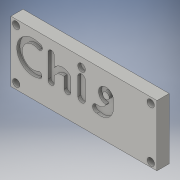
# Autodesk Inventor part: NewName
Saved by Autodesk Inventor 2016 (Build 200138000, 138)
## iProperties
Created: 2016-09-23
Part Number: NewName
Material: Generic
Document SubType Name: Modeling
Designer: Shaan Sharma
Density: 1 g/cm^3
Appearance: Default
Author: Shaan Sharma
Autodesk Inventor part; units mm, degrees
ref_plane "YZ Plane" through (0, 0, 0) normal (1, 0, 0) x (0, 1, 0)
ref_plane "XZ Plane" through (0, 0, 0) normal (0, 1, 0) x (-1, 0, 0)
ref_plane "XY Plane" through (0, 0, 0) normal (0, 0, 1) x (1, 0, 0)
sketch "Sketch1" plane through (0, 0, 0) normal (0, 0, 1) x (1, 0, 0)
  line L0 (-174.625, 111.125) -> (130.175, 111.125)
  line L1 (130.175, 111.125) -> (130.175, -15.875)
  line L2 (130.175, -15.875) -> (-174.625, -15.875)
  line L3 (-174.625, -15.875) -> (-174.625, 111.125)
  point P0 (0, 0)
  dimension "d0" = 127
  dimension "d1" = 304.8
  constraints: 8 end point, 2 parallel, 1 horizontal, 1 perpendicular
  measures "d0" distance of L2.end L0.start
  measures "d1" distance of L1.end L2.end
extrude "Extrusion1" add sketch "Sketch1" along normal blind 25.4
sketch "Sketch2" plane through (0, 0, 25.4) normal (0, 0, 1) x (1, 0, 0)
  arc A0 (-115.8875, 79.375) -> (-115.8875, 41.275) centre (-128.1906, 60.325) ccw
  arc A1 (-115.8875, 92.075) -> (-115.8875, 28.575) centre (-128.1906, 60.325) ccw
  arc A2 (-115.8875, 28.575) -> (-115.8875, 41.275) centre (-115.8875, 34.925) ccw
  arc A3 (-115.8875, 79.375) -> (-115.8875, 92.075) centre (-115.1373, 85.725) ccw
  line L0 (-96.8375, 36.5125) -> (-96.8375, 85.725)
  line L1 (-84.1375, 36.5125) -> (-84.1375, 85.725)
  arc A4 (-96.8375, 36.5125) -> (-84.1375, 36.5125) centre (-90.4875, 34.925) ccw
  arc A5 (-84.1375, 85.725) -> (-96.8375, 85.725) centre (-90.4875, 85.725) ccw
  arc A6 (-49.4641, 48.1659) -> (-84.1375, 49.1296) centre (-67.0914, 38.1936) ccw
  arc A7 (-49.2125, 63.5) -> (-84.1375, 63.5) centre (-66.675, 52.2579) ccw
  line L2 (-49.4641, 48.1659) -> (-49.4641, 34.7551)
  line L3 (-49.4641, 63.8815) -> (-49.4641, 48.1659)
  line L4 (-63.5, 34.7551) -> (-63.5, 72.7821)
  arc A8 (-63.5, 34.7551) -> (-49.4641, 34.7551) centre (-56.4821, 35.6136) ccw
  line L5 (-34.925, 35.6136) -> (-34.925, 72.7821)
  line L6 (-19.05, 35.6136) -> (-19.05, 72.7821)
  arc A9 (-34.925, 35.6136) -> (-19.05, 35.6136) centre (-26.9875, 36.5341) ccw
  arc A10 (-19.05, 72.7821) -> (-34.925, 72.7821) centre (-26.9875, 72.7821) ccw
  circle A11 centre (-26.9875, 92.075) radius 7.9375
  circle A12 centre (23.8125, 66.6933) radius 15.538
  circle A13 centre (23.8125, 66.6933) radius 6.8831
  arc A14 (5.1159, 25.5884) -> (39.3505, 51.137) centre (12.7, 51.137) ccw
  line L7 (39.3505, 51.137) -> (39.3505, 66.675)
  arc A15 (5.5549, 41.3745) -> (23.8166, 51.1553) centre (9.031, 56.8228) ccw
  arc A16 (5.5549, 41.3745) -> (5.1159, 25.5884) centre (3.7885, 33.5244) ccw
  point P0 (0, 0)
  constraints: 32 point on circle, 17 centre point, 16 end point, 8 vertical, 5 tangent, 2 point on line, 1 coincident, 1 concentric
emboss "Emboss1" sketch "Sketch2" operation cut depth 6.35 direction (0, 0, -1)
hole "Hole1" at (-163.3305, -4.0099, 25.4) direction (0, 0, -1) diameter 15.24 end through all
hole "Hole2" at (-163.7335, 100.3697, 25.4) direction (0, 0, -1) diameter 15.24 end through all
hole "Hole3" at (117.1647, 99.5637, 25.4) direction (0, 0, -1) diameter 15.24 end through all
hole "Hole4" at (117.5677, -6.025, 25.4) direction (0, 0, -1) diameter 15.24 end through all
body "Solid1"
